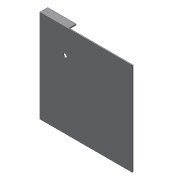
# Autodesk Inventor part: motor_mount_base1_template
Saved by Autodesk Inventor 2017 (Build 210142000, 142)
## iProperties
Created: 2018-10-29
Part Number: motor_mount_base1_template
Material: Generic
Document SubType Name: Modeling
Designer: mfans
Density: 1 g/cm^3
Appearance: Default
Author: mfans
Autodesk Inventor part; units mm, degrees
ref_plane "YZ Plane" through (0, 0, 0) normal (1, 0, 0) x (0, 1, 0)
ref_plane "XZ Plane" through (0, 0, 0) normal (0, 1, 0) x (-1, 0, 0)
ref_plane "XY Plane" through (0, 0, 0) normal (0, 0, 1) x (1, 0, 0)
sketch "Sketch1" plane through (0, 0, 0) normal (0, 1, 0) x (-1, 0, 0)
  line L0 (45, 45) -> (-45, 45)
  line L1 (-45, 45) -> (-45, -45)
  line L2 (-45, -45) -> (45, -45)
  line L3 (45, -45) -> (45, 45)
  line L4 (45, 45) -> (-45, -45) construction
  line L5 (-45, 45) -> (45, -45) construction
  line L6 (-46, 46) -> (46, 46)
  line L7 (46, 46) -> (46, -46)
  line L8 (46, -46) -> (-46, -46)
  line L9 (-46, -46) -> (-46, 46)
  line L10 (-46, 46) -> (46, -46) construction
  line L11 (46, 46) -> (-46, -46) construction
  point P0 (0, 0)
  dimension "d0" = 90
  dimension "d1" = 90
  dimension "d2" = 92
  dimension "d3" = 92
  constraints: 24 end point, 4 midpoint, 4 parallel, 2 horizontal, 2 perpendicular
  measures "d0" distance of L2.end L1.end
  measures "d1" distance of L0.end L1.end
  measures "d2" distance of L7.end L8.end
  measures "d3" distance of L8.end L6.start
extrude "Extrusion1" add sketch "Sketch1" along normal blind 1 contours L3 L2 L1 L0 | L6 L7 L8 L9
sketch "Sketch2" plane through (0, 1, 0) normal (0, 1, 0) x (1, 0, 0)
  line L0 (-46, -46) -> (46, -46) projected
  line L1 (46, -46) -> (46, 46) projected
  line L2 (46, 46) -> (-46, 46) projected
  line L3 (-46, 46) -> (-46, -46) projected
  line L4 (45, 45) -> (-45, 45)
  line L5 (-45, -20.5) -> (-45, -45)
  line L6 (-45, -45) -> (-17.75, -45)
  line L7 (45, -45) -> (45, 45)
  line L8 (45, 45) -> (-45, -45) construction
  line L9 (-45, 45) -> (45, -45) construction
  line L10 (-27.75, -30.5) -> (-17.75, -30.5)
  line L11 (-17.75, -30.5) -> (-17.75, -29.5)
  line L12 (-17.75, -29.5) -> (-27.75, -29.5)
  line L13 (-27.75, -29.5) -> (-27.75, -30.5)
  line L14 (-27.75, -30.5) -> (-26.75, -30.5)
  line L15 (-26.75, -30.5) -> (-26.75, -20.5)
  line L16 (-26.75, -20.5) -> (-27.75, -20.5)
  line L17 (-27.75, -20.5) -> (-27.75, -30.5)
  line L18 (-17.75, -45) -> (-17.75, -46)
  line L19 (-46, -46) -> (46, -46) projected
  line L20 (-45, -20.5) -> (-46, -20.5)
  point P0 (0, 0)
  dimension "d6" = 90
  dimension "d7" = 90
  dimension "d8" = 1
  dimension "d9" = 1
  dimension "d10" = 10
  dimension "d11" = 10
  dimension "d12" = 14.5
  dimension "d13" = 17.25
  constraints: 32 end point, 6 parallel, 4 perpendicular, 3 horizontal, 2 midpoint, 2 point on line, 1 vertical
  measures "d6" distance of L5.end L7.start
  measures "d7" distance of L4.end L5.end
  measures "d8" distance of L15.end L16.end
  measures "d9" distance of L10.end L11.end
  measures "d10" distance of L11.end L12.end
  measures "d11" distance of L14.end L15.end
  measures "d12" distance between parallel lines of L6 L10
  measures "d13" distance between parallel lines of L5 L17
sketch "Sketch3" plane through (0, 1, 0) normal (0, 1, 0) x (1, 0, 0)
  line L0 (-27.75, -30.5) -> (-17.75, -30.5) projected
  line L1 (-27.75, -20.5) -> (-27.75, -30.5) projected
  line L2 (-26.75, -30.5) -> (-26.75, -20.5) projected
  line L3 (-17.75, -29.5) -> (-27.75, -29.5) projected
  line L4 (-26.75, -20.5) -> (-27.75, -20.5) projected
  line L5 (-17.75, -45) -> (-17.75, -46) projected
  line L6 (-45, -20.5) -> (-46, -20.5) projected
  line L7 (-46, 46) -> (-46, -46) projected
  line L8 (-45, -20.5) -> (-46, -20.5)
  line L9 (-46, -20.5) -> (-46, -46)
  line L10 (-46, -46) -> (-45, -46)
  line L11 (-45, -46) -> (-45, -20.5)
  line L12 (-46, -46) -> (46, -46) projected
  line L13 (-46, -46) -> (-17.75, -46)
  line L14 (-17.75, -46) -> (-17.75, -45)
  line L15 (-17.75, -45) -> (-46, -45)
  line L16 (-46, -45) -> (-46, -46)
  line L17 (-27.75, -30.5) -> (-17.75, -30.5)
  line L18 (-17.75, -30.5) -> (-17.75, -29.5)
  line L19 (-17.75, -29.5) -> (-27.75, -29.5)
  line L20 (-27.75, -29.5) -> (-27.75, -30.5)
  point P0 (0, 0)
  constraints: 24 end point, 6 parallel, 3 horizontal, 3 perpendicular
extrude "Extrusion2" add sketch "Sketch3" along normal blind 7
sketch "Sketch4" plane through (-45, 1, 20.5) normal (0, 0, -1) x (-1, 0, 0)
  line L0 (-17.25, 0) -> (-18.25, 0) projected
  line L1 (-17.25, 0) -> (-17.25, 7) projected
  line L2 (-18.25, 7) -> (-17.25, 7) projected
  line L3 (-18.25, 0) -> (-18.25, 7) projected
  line L4 (1, 0) -> (0, 0) projected
  line L5 (1, 0) -> (1, 7) projected
  line L6 (0, 7) -> (1, 7) projected
  line L7 (0, 0) -> (0, 7) projected
  line L8 (0, 0) -> (-27.25, 0) projected
  arc A0 (-17.25, 4.027) -> (0, 4.027) centre (-8.625, 11.25) ccw
  line L9 (-91, 0) -> (1, 0) projected
  line L10 (-17.25, 0) -> (-17.25, 7) projected
  line L11 (-8.625, 0) -> (-17.25, 0)
  line L12 (-17.25, 0) -> (-17.25, 4.027)
  line L13 (0, 0) -> (0, 7) projected
  line L14 (-8.625, 0) -> (0, 0)
  line L15 (0, 0) -> (0, 4.027)
  point P0 (-45, -1)
  dimension "d16" = 22.5
  dimension "d17" = 8.625
  constraints: 8 end point, 3 point on circle, 3 point on line, 1 centre point, 1 tangent
  measures "d16" diameter of A0
  measures "d17" distance from line of L1 A0.centre
extrude "Extrusion3" add sketch "Sketch4" against normal blind 10 contours A0 L7 L8 | L1 A0 L8
sketch "Sketch5" plane through (0, 1, 0) normal (0, 1, 0) x (1, 0, 0)
  line L0 (-17.75, -46) -> (46, -46) projected
  line L1 (-46, -20.5) -> (-46, -46) projected
  point P0 (0, 0)
  point P1 (-21, -21)
  dimension "d23" = 25
  dimension "d24" = 25
  measures "d23" distance from line of L0 point (-21, -21)
  measures "d24" distance from line of L1 point (-21, -21)
hole "Hole1" at (-21, 1, 21) direction (0, -1, 0) diameter 4 end through all
body "Solid1"
